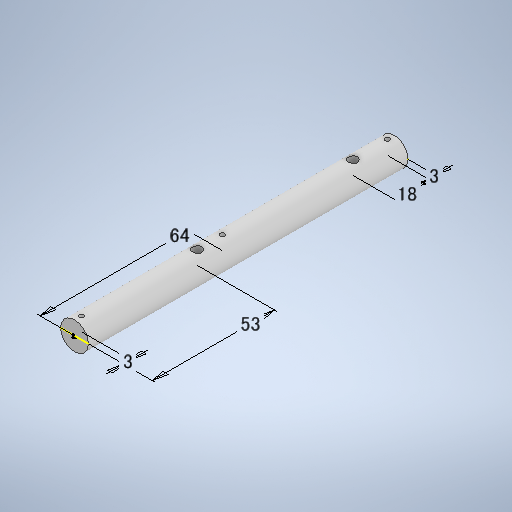
# Autodesk Inventor part: ローラー_軸
Saved by Autodesk Inventor 2025.1 (Build 291241020, 241B)
## iProperties
Created: 2024-10-14
Part Number: ローラー_軸
Material: 一般
Document SubType Name: Modeling
Designer: taiju
Density: 1 g/cm^3
Appearance: 既定
Author: taiju
Autodesk Inventor part; units mm, degrees
ref_plane "YZ Plane" through (0, 0, 0) normal (1, 0, 0) x (0, 1, 0)
ref_plane "XZ Plane" through (0, 0, 0) normal (0, 1, 0) x (-1, 0, 0)
ref_plane "XY Plane" through (0, 0, 0) normal (0, 0, 1) x (1, 0, 0)
sketch "スケッチ1" plane through (0, 0, 0) normal (0, 0, 1) x (1, 0, 0)
  circle A0 centre (0, 0) radius 6
  dimension "d0" = 12
  constraints: 1 centre point, 1 coincident
  measures "d0" diameter of A0
extrude "押し出し1" add sketch "スケッチ1" against normal blind 138.5
sketch "スケッチ2" plane through (0, 0, 0) normal (0, 1, 0) x (-1, 0, 0)
  line L0 (0, 0) -> (0, -138.5)
  line L1 (-6, -138.5) -> (6, -138.5) projected
  line L2 (6, 0) -> (-6, 0) projected
  point P0 (0, -3)
  point P1 (0, -53)
  point P2 (0, -64)
  point P3 (0, -120.5)
  point P4 (0, -135.5)
  dimension "d3" = 3
  dimension "d4" = 53
  dimension "d5" = 64
  dimension "d6" = 3
  dimension "d7" = 18
  constraints: 5 point on line, 2 end point, 2 midpoint
  measures "d3" distance from line of point (0, -3) L2
  measures "d4" distance from line of point (0, -53) L2
  measures "d5" distance of point (0, -64) point (0, 0)
  measures "d6" distance from line of point (0, -135.5) L1
  measures "d7" distance from line of point (0, -120.5) L1
hole "穴1" at (0, 0, -3) at (0, 0, -64) at (0, 0, -135.5) direction (0, -1, 0) diameter 2 end through all both
hole "穴2" at (0, 0, -53) at (0, 0, -120.5) direction (0, -1, 0) diameter 4 end through all both
